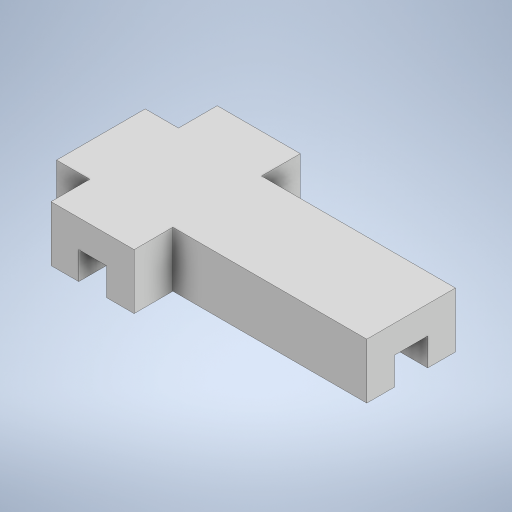
# Autodesk Inventor part: BTArm
Saved by Autodesk Inventor 2023 (Build 270158000, 158)
## iProperties
Created: 2023-04-18
Part Number: BTArm
Material: Generic
Document SubType Name: Modeling
Designer: Anders
Density: 1 g/cm^3
Appearance: Default
Author: Anders
Autodesk Inventor part; units mm, degrees
ref_plane "YZ Plane" through (0, 0, 0) normal (1, 0, 0) x (0, 1, 0)
ref_plane "XZ Plane" through (0, 0, 0) normal (0, 1, 0) x (-1, 0, 0)
ref_plane "XY Plane" through (0, 0, 0) normal (0, 0, 1) x (1, 0, 0)
sketch "Sketch1" plane through (0, 0, 0) normal (0, 1, 0) x (-1, 0, 0)
  line L0 (0, 0) -> (11, 0)
  line L1 (11, 0) -> (11, -6)
  line L2 (11, -6) -> (0, -6)
  line L3 (0, -6) -> (0, 0)
  line L4 (0, 0) -> (-5, 0)
  line L5 (-5, 0) -> (-5, 12)
  line L6 (-5, 12) -> (0, 12)
  line L7 (0, 12) -> (0, 0)
  line L8 (0, -6) -> (-5, -6)
  line L9 (-5, -6) -> (-5, -18)
  line L10 (-5, -18) -> (0, -18)
  line L11 (0, -18) -> (0, -6)
  line L12 (-5, -6) -> (-45, -6)
  line L13 (-45, -6) -> (-45, 0)
  line L14 (-45, 0) -> (-5, 0)
  line L15 (-5, 0) -> (-5, -6)
  line L16 (-5, -6) -> (-45, -6)
  line L17 (-45, -6) -> (-45, -11)
  line L18 (-45, -11) -> (-5, -11)
  line L19 (-5, -11) -> (-5, -6)
  line L20 (-5, 0) -> (-45, 0)
  line L21 (-45, 0) -> (-45, 5)
  line L22 (-45, 5) -> (-5, 5)
  line L23 (-5, 5) -> (-5, 0)
  line L24 (-5, 0) -> (-10, 0)
  line L25 (-10, 0) -> (-10, 12)
  line L26 (-10, 12) -> (-5, 12)
  line L27 (-5, 12) -> (-5, 0)
  line L28 (0, 0) -> (5, 0)
  line L29 (5, 0) -> (5, 12)
  line L30 (5, 12) -> (0, 12)
  line L31 (0, 12) -> (0, 0)
  line L32 (0, -6) -> (5, -6)
  line L33 (5, -6) -> (5, -18)
  line L34 (5, -18) -> (0, -18)
  line L35 (0, -18) -> (0, -6)
  line L36 (-5, -18) -> (-10, -18)
  line L37 (-10, -18) -> (-10, -6)
  line L38 (-10, -6) -> (-5, -6)
  line L39 (-5, -6) -> (-5, -18)
  line L40 (11, 0) -> (5, 0)
  line L41 (5, 0) -> (5, 5)
  line L42 (5, 5) -> (11, 5)
  line L43 (11, 5) -> (11, 0)
  line L44 (11, -6) -> (5, -6)
  line L45 (5, -6) -> (5, -11)
  line L46 (5, -11) -> (11, -11)
  line L47 (11, -11) -> (11, -6)
  point P0 (-10, -11)
  point P1 (-10, 5)
  dimension "d0" = 11
  dimension "d1" = 6
  dimension "d2" = 5
  dimension "d3" = 12
  dimension "d4" = 5
  dimension "d5" = 12
  dimension "d6" = 40
  dimension "d7" = 5
  dimension "d8" = 5
  dimension "d9" = 5
  dimension "d10" = 5
  dimension "d11" = 5
  dimension "d12" = 5
  constraints: 96 end point, 24 parallel, 12 horizontal, 12 perpendicular, 7 point on line
  measures "d0" distance of L1.end L2.end
  measures "d1" distance of L0.end L1.end
  measures "d2" distance of L5.end L6.end
  measures "d3" distance of L4.end L5.end
  measures "d4" distance of L10.end L9.end
  measures "d5" distance of L9.end L8.end
  measures "d6" distance of L13.end L14.end
  measures "d7" distance of L17.end L16.end
  measures "d8" distance of L20.end L21.end
  measures "d9" distance of L25.end L26.end
  measures "d10" distance of L33.end L34.end
  measures "d11" distance between parallel lines of L42 L0
  measures "d12" distance of L29.end L30.end
extrude "Extrusion1" add sketch "Sketch1" along normal blind 5 contours L7 L30 L29 L0 | L29 L42 L43 L0 | L2 L33 L34 L11 | L14 L25 L22 L5 | L2 L47 L46 L33 | L9 L18 L37 L12 | L22 L25 L26 L5 | L14 L21 L22 L25 | L9 L36 L37 L18 | L37 L18 L17 L12
sketch "Sketch2" plane through (0, 5, 0) normal (0, 1, 0) x (1, 0, 0)
  line L0 (-11, 6) -> (0, 6) projected
  line L1 (0, 6) -> (0, 18) projected
  line L2 (0, 18) -> (-5, 18) projected
  line L3 (-5, 18) -> (-5, 11) projected
  line L4 (-5, 11) -> (-11, 11) projected
  line L5 (-11, 11) -> (-11, 6) projected
  line L6 (5, 6) -> (45, 6) projected
  line L7 (45, 6) -> (45, 11) projected
  line L8 (45, 11) -> (10, 11) projected
  line L9 (10, 11) -> (10, 18) projected
  line L10 (10, 18) -> (5, 18) projected
  line L11 (5, 18) -> (5, 6) projected
  line L12 (10, -12) -> (10, -5) projected
  line L13 (10, -5) -> (45, -5) projected
  line L14 (45, -5) -> (45, 0) projected
  line L15 (45, 0) -> (5, 0) projected
  line L16 (5, 0) -> (5, -12) projected
  line L17 (5, -12) -> (10, -12) projected
  line L18 (-11, -5) -> (-5, -5) projected
  line L19 (-5, -5) -> (-5, -12) projected
  line L20 (-5, -12) -> (0, -12) projected
  line L21 (0, -12) -> (0, 0) projected
  line L22 (0, 0) -> (-11, 0) projected
  line L23 (-11, 0) -> (-11, -5) projected
  line L24 (-11, 11) -> (10, 11)
  line L25 (10, 11) -> (10, -5)
  line L26 (10, -5) -> (-11, -5)
  line L27 (-11, -5) -> (-11, 11)
  line L28 (-5, 18) -> (10, 18)
  line L29 (10, 18) -> (10, 11)
  line L30 (10, 11) -> (-5, 11)
  line L31 (-5, 11) -> (-5, 18)
  line L32 (-5, -5) -> (10, -5)
  line L33 (10, -5) -> (10, -12)
  line L34 (10, -12) -> (-5, -12)
  line L35 (-5, -12) -> (-5, -5)
  constraints: 24 end point, 6 parallel, 3 horizontal, 3 perpendicular
extrude "Extrusion2" add sketch "Sketch2" along normal blind 5 contours L5 L4 L24 L1 L0 | L0 L1 L24 L11 L6 L25 L15 L16 L26 L21 L22 L27 | L22 L21 L26 L18 L23 | L24 L3 L2 L1 | L1 L28 L11 L24 | L24 L25 L6 L11 | L11 L10 L9 L24 | L26 L16 L34 L21 | L21 L20 L19 L26 | L26 L12 L17 L16 | L16 L15 L25 L26
sketch "Sketch3" plane through (0, 5, 0) normal (0, 1, 0) x (1, 0, 0)
  point P0 (0, 0)
sketch "Sketch4" plane through (0, 5, 0) normal (0, 1, 0) x (1, 0, 0)
  line L0 (10, 0) -> (10, -5) projected
  line L1 (10, -5) -> (45, -5) projected
  line L2 (45, -5) -> (45, 0) projected
  line L3 (45, 0) -> (10, 0) projected
  line L4 (10, 11) -> (10, 6) projected
  line L5 (10, 6) -> (45, 6) projected
  line L6 (45, 6) -> (45, 11) projected
  line L7 (45, 11) -> (10, 11) projected
  point P0 (0, 0)
extrude "Extrusion3" add sketch "Sketch4" along normal blind 5
sketch "Sketch5" plane through (5, 0, -6) normal (0, 0, 1) x (1, 0, 0)
  line L0 (40, 0) -> (40, 10) projected
  line L1 (40, 0) -> (40, 10) projected
  line L2 (0, 0) -> (40, 0) projected
  line L3 (40, 0) -> (40, 10) projected
  line L4 (5, 10) -> (40, 10) projected
  line L5 (5, 5) -> (5, 10) projected
  line L6 (0, 5) -> (5, 5) projected
  line L7 (0, 0) -> (0, 5) projected
  line L8 (40, 10) -> (5, 10)
  line L9 (5, 10) -> (5, 5)
  line L10 (5, 5) -> (40, 5)
  line L11 (40, 5) -> (40, 10)
  point P0 (-5, 0)
  dimension "d19" = 5
  constraints: 8 end point, 2 parallel, 1 horizontal, 1 perpendicular
  measures "d19" distance of L5.start L8.end
extrude "Extrusion4" add sketch "Sketch5" along normal up to surface (6 mm away) contours L10 L5 L4 L0
body "Solid1"
